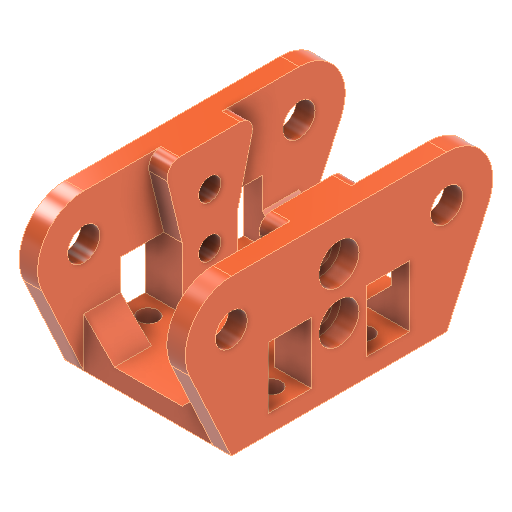
# Autodesk Inventor part: Y Axis Gantry Baseblock (CNC)
Saved by Autodesk Inventor 2023.2 (Build 272271000, 271)
## iProperties
Created: 2023-02-03
Part Number: Y Axis Gantry Baseblock (CNC)
Material: ABS Plastic
Document SubType Name: Modeling
Designer: remop
Density: 1.06 g/cm^3
Appearance: Smooth - Light Orange
Mass: 18.2849 g
Surface Area: 63.9276 cm^2
Volume: 6.77218 cm^3
Author: remop
Autodesk Inventor part; units mm, degrees
ref_plane "YZ Plane" through (0, 0, 0) normal (1, 0, 0) x (0, 1, 0)
ref_plane "XZ Plane" through (0, 0, 0) normal (0, 1, 0) x (-1, 0, 0)
ref_plane "XY Plane" through (0, 0, 0) normal (0, 0, 1) x (1, 0, 0)
sketch "Sketch8" plane through (0, 0, 0) normal (0, 1, 0) x (-1, 0, 0)
  line L0 (-13.5, -17.5) -> (13.5, -17.5)
  line L1 (13.5, -17.5) -> (13.5, 17.5)
  line L2 (13.5, 17.5) -> (-13.5, 17.5)
  line L3 (-13.5, 17.5) -> (-13.5, -17.5)
  line L4 (-13.5, -17.5) -> (13.5, 17.5) construction
  line L5 (13.5, -17.5) -> (-13.5, 17.5) construction
  circle A0 centre (10, -7.5) radius 1.6
  circle A1 centre (10, 7.5) radius 1.6
  circle A2 centre (-10, 7.5) radius 1.6
  circle A3 centre (-10, -7.5) radius 1.6
  point P0 (0, 0)
  dimension "d38" = 35
  dimension "d39" = 27
  dimension "d40" = 20
  dimension "d41" = 15
  dimension "d42" = 7.5
  dimension "d43" = 10
  dimension "d44" = 3.2
  constraints: 12 end point, 4 centre point, 3 equal radius, 2 horizontal alignment, 2 midpoint, 2 parallel, 2 vertical alignment, 1 horizontal, 1 perpendicular
  measures "d38" distance of L0.end L1.end
  measures "d39" distance of L1.end L2.end
  measures "d40" distance of A2.centre A1.centre
  measures "d41" distance of A1.centre A0.centre
  measures "d42" vertical distance of A1.centre point (0, 0)
  measures "d43" horizontal distance of A1.centre point (0, 0)
  measures "d44" diameter of A1
extrude "Extrusion7" add sketch "Sketch8" against normal blind 3
sketch "Sketch14" plane through (0, 0, 0) normal (0, 1, 0) x (1, 0, 0)
  line L0 (-13.5, 17.5) -> (-13.5, -17.5) projected
  line L1 (-13.5, -17.5) -> (13.5, -17.5) projected
  line L2 (13.5, -17.5) -> (13.5, 17.5) projected
  line L3 (13.5, 17.5) -> (-13.5, 17.5) projected
  circle A0 centre (-10, 7.5) radius 1.6 projected
  circle A1 centre (-10, -7.5) radius 1.6 projected
  circle A2 centre (10, -7.5) radius 1.6 projected
  circle A3 centre (10, 7.5) radius 1.6 projected
  line L4 (13.5, -17.5) -> (13.5, 17.5) projected
  line L5 (13.5, 4.5) -> (7.5, 4.5)
  line L6 (7.5, 4.5) -> (7.5, -4.5)
  line L7 (7.5, -4.5) -> (13.5, -4.5)
  line L8 (13.5, -4.5) -> (13.5, 4.5)
  point P0 (0, 0)
  dimension "d79" = 7.5
  dimension "d80" = 3
  dimension "d81" = 3
  constraints: 8 end point, 2 parallel, 1 horizontal, 1 perpendicular, 1 point on line
  measures "d79" distance from line of point (0, 0) L6
  measures "d80" distance from line of A3.centre L5
  measures "d81" distance from line of A2.centre L7
extrude "Extrusion12" add sketch "Sketch14" along normal blind 22.3 contours L2 L7 L6 L5
sketch "Sketch15" plane through (13.5, -3, 17.5) normal (1, 0, 0) x (0, 0, -1)
  line L0 (0, 3) -> (13, 3) projected
  line L1 (0, 3) -> (0, 0) projected
  line L2 (35, 0) -> (0, 0) projected
  line L3 (35, 3) -> (35, 0) projected
  line L4 (22, 3) -> (35, 3) projected
  line L5 (22, 3) -> (22, 25.3) projected
  line L6 (13, 25.3) -> (22, 25.3) projected
  line L7 (13, 3) -> (13, 25.3) projected
  line L8 (35, 3) -> (35, 0) projected
  line L9 (35, 0) -> (41.8017, 14.6399)
  circle A0 centre (35, 17.8) radius 2.6
  circle A1 centre (35, 17.8) radius 7.5
  circle A2 centre (0, 17.8) radius 2.6
  circle A3 centre (0, 17.8) radius 7.5
  line L10 (-275, -9) -> (225, -9) projected
  line L11 (0, 0) -> (-6.8017, 14.6399)
  line L12 (0, 25.3) -> (35, 25.3)
  point P0 (17.5, 3)
  point P1 (13, 25.3)
  point P2 (22, 25.3)
  dimension "d84" = 5.2
  dimension "d85" = 35
  dimension "d86" = 17.5
  dimension "d87" = 26.8
  dimension "d88" = 15
  constraints: 6 end point, 4 centre point, 4 point on circle, 4 tangent, 2 coincident, 2 equal radius, 1 horizontal alignment
  measures "d84" diameter of A0
  measures "d85" distance of A2.centre A0.centre
  measures "d86" horizontal distance of point (17.5, 3) A2.centre
  measures "d87" distance from line of A0.centre L10
  measures "d88" diameter of A1
extrude "Extrusion13" add sketch "Sketch15" against normal blind 3 contours L1 L11 A3 L12 L7 L0 | L3 L4 L5 L12 A1 L9 | A3 | A1
sketch "Sketch16" plane through (10.5, -3, 17.5) normal (-1, 0, 0) x (0, 0, 1)
  arc A0 (-35, 25.3) -> (-41.8017, 14.6399) centre (-35, 17.8) ccw projected
  line L0 (-41.8017, 14.6399) -> (-35, 0) projected
  line L1 (-35, 3) -> (-35, 0) projected
  line L2 (-26.5199, 3) -> (-35, 3) projected
  line L3 (-26.5199, 3) -> (-23.4801, 3) projected
  line L4 (-22, 3) -> (-23.4801, 3) projected
  line L5 (-22, 25.3) -> (-22, 3) projected
  line L6 (-22, 25.3) -> (-35, 25.3) projected
  circle A1 centre (-35, 17.8) radius 2.6 projected
  arc A2 (6.8017, 14.6399) -> (0, 25.3) centre (0, 17.8) ccw projected
  line L7 (0, 25.3) -> (-13, 25.3) projected
  line L8 (-13, 3) -> (-13, 25.3) projected
  line L9 (-11.5199, 3) -> (-13, 3) projected
  line L10 (-11.5199, 3) -> (-8.4801, 3) projected
  line L11 (0, 3) -> (-8.4801, 3) projected
  line L12 (0, 0) -> (0, 3) projected
  line L13 (0, 0) -> (6.8017, 14.6399) projected
  circle A3 centre (0, 17.8) radius 2.6 projected
  line L14 (-22, 3) -> (-29, 3)
  line L15 (-29, 3) -> (-29, 13)
  line L16 (-29, 13) -> (-22, 13)
  line L17 (-22, 13) -> (-22, 3)
  line L18 (-11.5199, 3) -> (-13, 3) projected
  line L19 (-13, 3) -> (-6, 3)
  line L20 (-6, 3) -> (-6, 13)
  line L21 (-6, 13) -> (-13, 13)
  line L22 (-13, 13) -> (-13, 3)
  line L23 (-23.4, 0) -> (-26.6, 0) projected
  line L24 (-26.6, 3) -> (-23.4, 3) projected
  line L25 (-8.4, 0) -> (-11.6, 0) projected
  line L26 (-11.6, 3) -> (-8.4, 3) projected
  point P0 (-17.5, 3)
  point P1 (-10, 0)
  point P2 (-6, 3)
  dimension "d91" = 7
  dimension "d92" = 3
  dimension "d93" = 10
  constraints: 16 end point, 4 parallel, 2 equal length, 2 horizontal, 2 perpendicular, 1 midpoint
  measures "d91" distance of L15.end L16.end
  measures "d92" distance from line of L8 point (-10, 0)
  measures "d93" distance of L14.end L15.end
extrude "Extrusion14" cut sketch "Sketch16" against normal blind 22.3 contours L5 L4 L3 L2 L15 L16 | L21 L20 L11 L10 L9 L8
sketch "Sketch17" plane through (10.5, -3, 17.5) normal (-1, 0, 0) x (0, 0, 1)
  circle A0 centre (-35, 17.8) radius 2.6 projected
  line L0 (-29, 3) -> (-29, 13) projected
  line L1 (-29, 13) -> (-22, 13) projected
  line L2 (-22, 25.3) -> (-22, 13) projected
  line L3 (-22, 25.3) -> (-35, 25.3) projected
  arc A1 (-35, 25.3) -> (-41.8017, 14.6399) centre (-35, 17.8) ccw projected
  line L4 (-41.8017, 14.6399) -> (-35, 0) projected
  line L5 (-35, 3) -> (-35, 0) projected
  line L6 (-29, 3) -> (-35, 3) projected
  circle A2 centre (0, 17.8) radius 2.6 projected
  line L7 (-13, 13) -> (-6, 13) projected
  line L8 (-6, 13) -> (-6, 3) projected
  line L9 (0, 3) -> (-6, 3) projected
  line L10 (0, 0) -> (0, 3) projected
  line L11 (0, 0) -> (6.8017, 14.6399) projected
  arc A3 (6.8017, 14.6399) -> (0, 25.3) centre (0, 17.8) ccw projected
  line L12 (0, 25.3) -> (-13, 25.3) projected
  line L13 (-13, 13) -> (-13, 25.3) projected
  line L14 (-13, 13) -> (-10, 25.3)
  line L15 (-22, 13) -> (-25, 25.3)
  line L16 (-35, 25.3) -> (0, 25.3) projected
  point P0 (-17.5, 3)
  dimension "d96" = 15
  constraints: 4 end point, 2 point on line, 1 equal length
  measures "d96" distance of L14.end L15.end
extrude "Extrusion15" add sketch "Sketch17" along normal up to surface (3 mm away) contours L12 L14 L13 | L15 L3 L2
fillet "Fillet2" radius 2 2 edges at (9, 22.3, -7.5) (9, 22.3, 7.5)
mirror "Mirror1" about plane through (0, 0, 0) normal (1, 0, 0) of "Extrusion12", "Extrusion13", "Extrusion14", "Extrusion15", "Fillet2"
chamfer "Chamfer1" distance 5 angle 45 4 edges at (-10.5, 0, 14.5) (-10.5, 0, -14.5) (10.5, 0, 14.5) (10.5, 0, -14.5)
sketch "Sketch18" plane through (-13.5, 22.3, -17.5) normal (-1, 0, 0) x (0, 0, 1)
  line L0 (13, -22.3) -> (6, -22.3) projected
  line L1 (6, -22.3) -> (6, -12.3) projected
  line L2 (6, -12.3) -> (13, -12.3) projected
  line L3 (13, -12.3) -> (13, -22.3) projected
  line L4 (29, -22.3) -> (22, -22.3) projected
  line L5 (22, -22.3) -> (22, -12.3) projected
  line L6 (22, -12.3) -> (29, -12.3) projected
  line L7 (29, -12.3) -> (29, -22.3) projected
  circle A0 centre (0, -7.5) radius 2.6 projected
  circle A1 centre (35, -7.5) radius 2.6 projected
  line L8 (41.8017, -10.6601) -> (35, -25.3) projected
  arc A2 (41.8017, -10.6601) -> (35, 0) centre (35, -7.5) ccw projected
  line L9 (0, 0) -> (35, 0) projected
  arc A3 (0, 0) -> (-6.8017, -10.6601) centre (0, -7.5) ccw projected
  line L10 (0, -25.3) -> (-6.8017, -10.6601) projected
  line L11 (35, -25.3) -> (0, -25.3) projected
  point P0 (17.5, -22.3)
  point P1 (17.5, -7)
  point P2 (17.5, -15.3)
  dimension "d103" = 7
  dimension "d104" = 10
  measures "d103" distance from line of L9 point (17.5, -7)
  measures "d104" distance from line of L11 point (17.5, -15.3)
hole "Hole3" at (-13.5, 15.3, 0) at (-13.5, 7, 0) direction (1, 0, 0) diameter 3.6 end through all clearance for "Slotted Cheese Head Screw ISO 1207" size "M3" standard "ISO"
sketch "Sketch19" plane through (13.5, 22.3, 17.5) normal (1, 0, 0) x (0, 0, -1)
  circle A0 centre (17.5, -15.3) radius 1.8 projected
  circle A1 centre (17.5, -7) radius 1.8 projected
  circle A2 centre (17.5, -15.3) radius 3.25
  circle A3 centre (17.5, -7) radius 3.25
  point P0 (17.5, -22.3)
  dimension "d112" = 6.5
  constraints: 2 centre point, 2 coincident, 1 equal radius
  measures "d112" diameter of A2
extrude "Extrusion16" cut sketch "Sketch19" against normal blind 3 contours A0 | A1 | A2 | A3
sketch "Sketch20" plane through (-13.5, 22.3, -17.5) normal (-1, 0, 0) x (0, 0, 1)
  circle A0 centre (17.5, -15.3) radius 3.25 projected
  circle A1 centre (17.5, -7) radius 3.25 projected
  point P0 (17.5, -22.3)
extrude "Extrusion17" cut sketch "Sketch20" against normal blind 3
equation "\"d42\" = 0.5 * d41"
equation "\"d43\" = 0.5 * d40"
equation "\"d81\" = d80"
equation "\"d86\" = 0.5 * d85"
body "Solid2"
